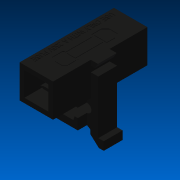
# Autodesk Inventor part: Soanar Power Module Fuse Cover
Saved by Autodesk Inventor 2016 (Build 200138000, 138)
## iProperties
Created: 2013-08-06
Material: ABS Plastic
Document SubType Name: Modeling
Designer: sdarley
Density: 1.06 g/cm^3
Appearance: Smooth - Black
Project: Power Entry Module - Soanar PP4003
Description: Soanar Power Module Fuse Cover
Author: sdarley
Title: Soanar Power Module Fuse Cover
Revision Number: 1
Autodesk Inventor part; units mm, degrees
ref_plane "YZ Plane" through (0, 0, 0) normal (1, 0, 0) x (0, 1, 0)
ref_plane "XZ Plane" through (0, 0, 0) normal (0, 1, 0) x (-1, 0, 0)
ref_plane "XY Plane" through (0, 0, 0) normal (0, 0, 1) x (1, 0, 0)
sketch "Sketch1" plane through (0, 0, 0) normal (0, 0, 1) x (1, 0, 0)
  line L0 (-3.05, -3.0141) -> (3.05, -3.0141)
  line L1 (3.05, 3.0141) -> (-3.05, 3.0141)
  line L2 (-3.05, 3.0141) -> (-3.05, -3.0141)
  line L3 (-3.05, -3.0141) -> (3.05, 3.0141) construction
  line L4 (3.05, -3.0141) -> (-3.05, 3.0141) construction
  line L5 (-4.25, -4.2) -> (4.25, -4.2)
  line L6 (4.25, -4.2) -> (4.25, 4.2)
  line L7 (4.25, 4.2) -> (-4.25, 4.2)
  line L8 (-4.25, 4.2) -> (-4.25, -4.2)
  line L9 (-4.25, -4.2) -> (4.25, 4.2) construction
  line L10 (4.25, -4.2) -> (-4.25, 4.2) construction
  line L11 (3.05, 1.3359) -> (2.2, 1.3359)
  line L12 (3.05, 1.9859) -> (2.2, 1.9859)
  arc A0 (2.2, 1.9859) -> (0.95, 1.6609) centre (2.2, -0.5805) ccw
  arc A1 (0.95, 1.6609) -> (2.2, 1.3359) centre (2.2, 3.9022) ccw
  line L13 (3.05, -3.0141) -> (3.05, 1.3359)
  line L14 (3.05, 1.9859) -> (3.05, 3.0141)
  point P0 (0, 0)
  dimension "d0" = 8.5
  dimension "d1" = 8.4
  dimension "d2" = 6.1
  dimension "d3" = 4.35
  dimension "d4" = 0.65
  dimension "d5" = 2.1
  dimension "d6" = 0.85
  constraints: 30 end point, 6 parallel, 5 perpendicular, 4 midpoint, 4 point on circle, 2 centre point, 2 horizontal, 2 tangent, 2 vertical alignment, 1 equal radius, 1 point on line
  measures "d0" distance between parallel lines of L6 L8
  measures "d1" distance between parallel lines of L5 L7
  measures "d2" distance between parallel lines of L13 L2
  measures "d3" distance between parallel lines of L0 L11
  measures "d4" distance between parallel lines of L11 L12
  measures "d5" distance from line of A0.end L14
  measures "d6" distance of L11.start L11.end
extrude "Extrusion1" add sketch "Sketch1" along normal mid plane 24
sketch "Sketch2" plane through (0, 0, 0) normal (0, 0, 1) x (1, 0, 0)
  line L0 (-3.05, 3.0141) -> (-3.05, -3.0141) projected
  line L1 (-3.05, -3.0141) -> (3.05, -3.0141) projected
  line L2 (3.05, -3.0141) -> (3.05, 1.3359) projected
  line L3 (3.05, 1.3359) -> (2.2, 1.3359) projected
  arc A0 (0.95, 1.6609) -> (2.2, 1.3359) centre (2.2, 3.9022) ccw projected
  arc A1 (2.2, 1.9859) -> (0.95, 1.6609) centre (2.2, -0.5805) ccw projected
  line L4 (2.2, 1.9859) -> (3.05, 1.9859) projected
  line L5 (3.05, 1.9859) -> (3.05, 3.0141) projected
  line L6 (3.05, 3.0141) -> (-3.05, 3.0141) projected
  line L7 (4.25, -4.2) -> (-4.25, -4.2) projected
  line L8 (-4.25, -4.2) -> (-4.25, 4.2) projected
  line L9 (-4.25, 4.2) -> (4.25, 4.2) projected
  line L10 (4.25, 4.2) -> (4.25, -4.2) projected
  line L11 (4.25, 1.45) -> (6.15, 1.45)
  line L12 (6.15, 1.45) -> (6.15, -12.1)
  line L13 (6.15, -12.1) -> (7.55, -12.1)
  line L14 (7.55, -12.1) -> (7.55, -14.2)
  line L15 (7.55, -14.2) -> (6.3, -14.2)
  line L16 (6.3, -14.2) -> (4.15, -12.25)
  line L17 (4.15, -12.25) -> (4.15, -11.2)
  line L18 (4.15, -11.2) -> (3.35, -10.7)
  line L19 (3.35, -10.7) -> (-4.25, -10.7)
  line L20 (-4.25, -10.7) -> (-4.25, -9.15)
  line L21 (-4.25, -9.15) -> (-1.15, -8.65)
  line L22 (-1.15, -8.65) -> (-1.15, -9)
  line L23 (-1.15, -9) -> (2.1, -9)
  line L24 (2.1, -9) -> (2.45, -8)
  line L25 (2.45, -8) -> (3.25, -8)
  arc A2 (3.25, -8) -> (3.25, -5.7) centre (3.25, -6.85) ccw
  line L26 (3.25, -5.7) -> (2.45, -5.7)
  arc A3 (2.45, -5.7) -> (1.8, -5.05) centre (1.8, -5.7) ccw
  line L27 (1.8, -5.05) -> (-1.15, -5.05)
  line L28 (-1.15, -5.05) -> (-1.15, -5.9)
  line L29 (-1.15, -5.9) -> (-4.25, -5)
  line L30 (-4.25, -5) -> (-4.25, -4.2)
  line L31 (-4.25, -4.2) -> (4.25, -4.2)
  line L32 (4.25, 1.45) -> (4.25, -4.2)
  line L33 (4.25, 4.2) -> (6.05, 4.2)
  line L34 (6.05, 4.2) -> (5.25, 2.85)
  line L35 (5.25, 2.85) -> (4.25, 2.85)
  line L36 (4.25, 4.2) -> (4.25, 2.85)
  point P0 (0, 0)
  dimension "d13" = 15.65
  dimension "d14" = 2.1
  dimension "d15" = 10.4
  dimension "d16" = 3.4
  dimension "d17" = 2
  dimension "d18" = 1.95
  dimension "d19" = 1.55
  dimension "d20" = 0.5
  dimension "d21" = 1.55
  dimension "d22" = 2.15
  dimension "d23" = 0.8
  dimension "d24" = 11.8
  dimension "d25" = 3.1
  dimension "d26" = 1.7
  dimension "d27" = 2.05
  dimension "d28" = 1.75
  dimension "d29" = 3.25
  dimension "d30" = 1
  dimension "d31" = 0.8
  dimension "d32" = 3.1
  dimension "d33" = 1.7
  dimension "d34" = 9.25
  dimension "d35" = 3.6
  dimension "d36" = 2.3
  dimension "d39" = 2.75
  dimension "d40" = 1.8
  dimension "d41" = 1
  dimension "d42" = 1.35
  constraints: 52 end point, 11 parallel, 4 perpendicular, 4 point on circle, 3 collinear, 2 centre point, 2 point on line, 2 tangent, 2 vertical alignment, 1 line through centre, 1 vertical
  measures "d13" distance between parallel lines of L15 L11
  measures "d14" distance between parallel lines of L15 L13
  measures "d15" distance between parallel lines of L8 L12
  measures "d16" distance between parallel lines of L14 L17
  measures "d17" distance between parallel lines of L12 L17
  measures "d18" distance from line of L16.end L15
  measures "d19" distance from line of L16.end L19
  measures "d20" distance from line of L17.end L19
  measures "d21" distance of L19.end L20.end
  measures "d22" distance from line of L15.end L17
  measures "d23" distance from line of L18.end L17
  measures "d24" distance between parallel lines of L14 L20
  measures "d25" distance from line of L21.end L20
  measures "d26" distance between parallel lines of L19 L23
  measures "d27" distance from line of L19 L21.end
  measures "d28" distance edge to line of A2 L12
  measures "d29" distance of L22.end L23.end
  measures "d30" distance between parallel lines of L23 L25
  measures "d31" distance from line of L29.end L7
  measures "d32" distance from line of L28.end L30
  measures "d33" distance from line of L7 L28.end
  measures "d34" distance between parallel lines of L9 L27
  measures "d35" horizontal distance of L28.end L26.end
  measures "d36" distance between parallel lines of L25 L26
  measures "d39" distance between parallel lines of L9 L11
  measures "d40" distance of L9.end L33.end
  measures "d41" distance of L34.end L35.end
  measures "d42" distance between parallel lines of L35 L33
extrude "Extrusion2" add sketch "Sketch2" along normal mid plane 4.8
sketch "Sketch3" plane through (0, 0, 2.4) normal (0, 0, 1) x (1, 0, 0)
  line L0 (-4.25, -4.2) -> (4.25, -4.2) projected
  line L1 (-4.25, -4.2) -> (-4.25, -5) projected
  line L2 (-4.25, -5) -> (-1.15, -5.9) projected
  line L3 (-1.15, -5.9) -> (-1.15, -5.05) projected
  line L4 (-1.15, -5.05) -> (1.8, -5.05) projected
  arc A0 (2.45, -5.7) -> (1.8, -5.05) centre (1.8, -5.7) ccw projected
  line L5 (2.45, -5.7) -> (3.25, -5.7) projected
  line L6 (3.25, -8) -> (2.45, -8) projected
  line L7 (2.45, -8) -> (2.1, -9) projected
  line L8 (2.1, -9) -> (-1.15, -9) projected
  line L9 (-1.15, -9) -> (-1.15, -8.65) projected
  line L10 (-1.15, -8.65) -> (-4.25, -9.15) projected
  line L11 (-4.25, -9.15) -> (-4.25, -10.7) projected
  line L12 (-4.25, -10.7) -> (3.35, -10.7) projected
  line L13 (3.25, -4.2) -> (3.25, -5.7)
  line L14 (3.25, -8) -> (3.25, -10.7)
  point P0 (0, 0)
  dimension "d43" = 7.5
  constraints: 4 end point, 4 point on line, 2 perpendicular, 1 vertical alignment
  measures "d43" distance between parallel lines of L14 L11
extrude "Extrusion3" add sketch "Sketch3" along normal blind 2.3
sketch "Sketch4" plane through (0, 0, -2.4) normal (0, 0, -1) x (-1, 0, 0)
  line L0 (-3.35, -10.7) -> (4.25, -10.7) projected
  line L1 (4.25, -10.7) -> (4.25, -9.15) projected
  line L2 (4.25, -9.15) -> (1.15, -8.65) projected
  line L3 (1.15, -8.65) -> (1.15, -9) projected
  line L4 (1.15, -9) -> (-2.1, -9) projected
  line L5 (-2.1, -9) -> (-2.45, -8) projected
  line L6 (-2.45, -8) -> (-3.25, -8) projected
  line L7 (-3.25, -5.7) -> (-2.45, -5.7) projected
  arc A0 (-1.8, -5.05) -> (-2.45, -5.7) centre (-1.8, -5.7) ccw projected
  line L8 (-1.8, -5.05) -> (1.15, -5.05) projected
  line L9 (1.15, -5.05) -> (1.15, -5.9) projected
  line L10 (1.15, -5.9) -> (4.25, -5) projected
  line L11 (4.25, -5) -> (4.25, -4.2) projected
  line L12 (-4.25, -4.2) -> (4.25, -4.2) projected
  line L13 (-3.25, -4.2) -> (-3.25, -5.7) projected
  line L14 (-3.25, -8) -> (-3.25, -10.7) projected
  point P0 (0, 0)
extrude "Extrusion4" add sketch "Sketch4" along normal blind 2.3
sketch "Sketch8" plane through (-4.25, 4.2, -12) normal (0, 1, 0) x (1, 0, 0)
  line L0 (8.5, 0) -> (8.5, -9.6) projected
  line L1 (0, 0) -> (8.5, 0) projected
  line L2 (6.575, -9.05) -> (6.575, -15.85)
  line L3 (3.575, -15.85) -> (3.575, -9.05)
  arc A0 (3, -8.475) -> (3.575, -9.05) centre (3.575, -8.475) ccw
  arc A1 (6.575, -9.05) -> (7.15, -8.475) centre (6.575, -8.475) ccw
  line L4 (3, -8.475) -> (3, -6.225)
  line L5 (3, -6.225) -> (4.025, -5.2)
  line L6 (4.025, -5.2) -> (6.125, -5.2)
  line L7 (6.125, -5.2) -> (7.15, -6.225)
  line L8 (7.15, -6.225) -> (7.15, -8.475)
  line L9 (3, -16.425) -> (3, -18.675)
  line L10 (3, -18.675) -> (4.025, -19.7)
  line L11 (4.025, -19.7) -> (6.125, -19.7)
  line L12 (6.125, -19.7) -> (7.15, -18.675)
  line L13 (7.15, -18.675) -> (7.15, -16.425)
  arc A2 (3.575, -15.85) -> (3, -16.425) centre (3.575, -16.425) ccw
  arc A3 (7.15, -16.425) -> (6.575, -15.85) centre (6.575, -16.425) ccw
  line L14 (4.025, -8.95) -> (6.125, -8.95)
  line L15 (6.125, -8.95) -> (6.125, -15.95)
  line L16 (6.125, -15.95) -> (4.025, -15.95)
  line L17 (4.025, -15.95) -> (4.025, -8.95)
  line L18 (4.2114, -5.65) -> (5.9386, -5.65)
  line L19 (5.9386, -5.65) -> (6.7, -6.4114)
  line L20 (6.7, -6.4114) -> (6.7, -8.5)
  line L21 (6.7, -8.5) -> (3.45, -8.5)
  line L22 (3.45, -8.5) -> (3.45, -6.4114)
  line L23 (3.45, -6.4114) -> (4.2114, -5.65)
  line L24 (3.45, -18.4886) -> (3.45, -16.4)
  line L25 (3.45, -16.4) -> (6.7, -16.4)
  line L26 (6.7, -16.4) -> (6.7, -18.4886)
  line L27 (6.7, -18.4886) -> (5.9386, -19.25)
  line L28 (5.9386, -19.25) -> (4.2114, -19.25)
  line L29 (4.2114, -19.25) -> (3.45, -18.4886)
  point P0 (4.25, -12)
  point P1 (5.075, -5.2)
  point P2 (5.075, -19.7)
  point P3 (5.075, -5.65)
  point P4 (5.075, -8.5)
  point P5 (5.075, -16.4)
  point P6 (5.075, -19.25)
  dimension "d90" = 14.5
  dimension "d91" = 1.35
  dimension "d92" = 4.15
  dimension "d93" = 3
  dimension "d95" = 6.8
  dimension "d96" = 2.1
  dimension "d97" = 5.2
  dimension "d104" = 7
  dimension "d105" = 0.45
  dimension "d106" = 0.45
  dimension "d107" = 0.45
  dimension "d108" = 0.45
  dimension "d109" = 0.45
  dimension "d110" = 0.45
  dimension "d111" = 0.45
  dimension "d112" = 0.45
  dimension "d113" = 0.45
  dimension "d114" = 0.45
  constraints: 56 end point, 16 parallel, 9 perpendicular, 8 point on circle, 7 vertical alignment, 6 midpoint, 5 horizontal alignment, 4 centre point, 4 equal length, 4 line through centre, 3 tangent, 1 collinear, 1 equal radius, 1 horizontal, 1 vertical
  measures "d90" distance between parallel lines of L11 L6
  measures "d91" distance between parallel lines of L0 L8
  measures "d92" distance between parallel lines of L8 L4
  measures "d93" distance between parallel lines of L2 L3
  measures "d95" distance of L3.start L3.end
  measures "d96" distance of L5.end L6.end
  measures "d97" distance between parallel lines of L1 L6
  measures "d104" distance between parallel lines of L16 L14
  measures "d105" distance between parallel lines of L2 L15
  measures "d106" distance between parallel lines of L17 L3
  measures "d107" distance between parallel lines of L5 L23
  measures "d108" distance between parallel lines of L8 L20
  measures "d109" distance between parallel lines of L6 L18
  measures "d110" distance between parallel lines of L21 L14
  measures "d111" distance between parallel lines of L11 L28
  measures "d112" distance between parallel lines of L13 L26
  measures "d113" distance between parallel lines of L12 L27
  measures "d114" distance between parallel lines of L16 L25
extrude "Extrusion8" cut sketch "Sketch8" against normal blind 0.1
sketch "Sketch5" plane through (-4.25, 4.2, -12) normal (0, 1, 0) x (1, 0, 0)
  line L0 (0, 0) -> (0, -24) projected
  line L1 (1.85, -1.3407) -> (1.85, -22.6593) construction
  line L2 (1.85, -22.6593) -> (0.5, -22.6593) construction
  line L3 (0.5, -22.6593) -> (0.5, -1.3407) construction
  line L4 (0.5, -1.3407) -> (1.85, -1.3407) construction
  line L5 (1.8278, -2.1206) -> (1.8278, -2.2557)
  line L6 (1.8278, -2.2557) -> (1.1058, -2.2557)
  spline S0 degree 2 poles (1.1058, -2.2557) (0.9243, -2.2557) (0.6917, -2.1853) (0.5566, -1.999) (0.5566, -1.8551) knots 0 0 0 1 2 3 3 3
  spline S1 degree 2 poles (0.5566, -1.8551) (0.5566, -1.6524) (0.7988, -1.4507) (1.1058, -1.4507) knots 0 0 0 1 2 2 2
  line L7 (1.1058, -1.4507) -> (1.8278, -1.4507)
  line L8 (1.8278, -1.4507) -> (1.8278, -1.5858)
  line L9 (1.8278, -1.5858) -> (1.1068, -1.5858)
  spline S2 degree 2 poles (1.1068, -1.5858) (0.9369, -1.5858) (0.7853, -1.6389) (0.7062, -1.7586) (0.7062, -1.8455) knots 0 0 0 1 2 3 3 3
  spline S3 degree 2 poles (0.7062, -1.8455) (0.7062, -1.9903) (0.8703, -2.1206) (1.1068, -2.1206) knots 0 0 0 1 2 2 2
  line L10 (1.1068, -2.1206) -> (1.8278, -2.1206)
  line L11 (0.9803, -2.4391) -> (0.9938, -2.5675)
  spline S4 degree 2 poles (0.9938, -2.5675) (0.8905, -2.5781) (0.7757, -2.6505) (0.7062, -2.7847) (0.7062, -2.8696) knots 0 0 0 1 2 3 3 3
  spline S5 degree 2 poles (0.7062, -2.8696) (0.7062, -2.9903) (0.8239, -3.1244) (0.9185, -3.1244) knots 0 0 0 1 2 2 2
  spline S6 degree 2 poles (0.9185, -3.1244) (0.9736, -3.1244) (1.0556, -3.0762) (1.1087, -2.9777) (1.1569, -2.8146) knots 0 0 0 1 2 3 3 3
  spline S7 degree 2 poles (1.1569, -2.8146) (1.2004, -2.6698) (1.2873, -2.5472) (1.4214, -2.4787) (1.5054, -2.4787) knots 0 0 0 1 2 3 3 3
  spline S8 degree 2 poles (1.5054, -2.4787) (1.6569, -2.4787) (1.85, -2.6746) (1.85, -2.8407) knots 0 0 0 1 2 2 2
  spline S9 degree 2 poles (1.85, -2.8407) (1.85, -2.9555) (1.7593, -3.1264) (1.5903, -3.221) (1.4764, -3.2248) knots 0 0 0 1 2 3 3 3
  line L12 (1.4764, -3.2248) -> (1.4649, -3.0945)
  spline S10 degree 2 poles (1.4649, -3.0945) (1.5865, -3.0839) (1.7042, -2.9584) (1.7042, -2.8455) knots 0 0 0 1 2 2 2
  spline S11 degree 2 poles (1.7042, -2.8455) (1.7042, -2.7306) (1.601, -2.609) (1.5189, -2.609) knots 0 0 0 1 2 2 2
  spline S12 degree 2 poles (1.5189, -2.609) (1.4436, -2.609) (1.4021, -2.6534) knots 0 0 0 1 1 1
  spline S13 degree 2 poles (1.4021, -2.6534) (1.3597, -2.6978) (1.3172, -2.8532) knots 0 0 0 1 1 1
  spline S14 degree 2 poles (1.3172, -2.8532) (1.2747, -3.0047) (1.2438, -3.0665) knots 0 0 0 1 1 1
  spline S15 degree 2 poles (1.2438, -3.0665) (1.1965, -3.1602) (1.0402, -3.2557) (0.932, -3.2557) knots 0 0 0 1 2 2 2
  spline S16 degree 2 poles (0.932, -3.2557) (0.8249, -3.2557) (0.6483, -3.1553) (0.5566, -2.9816) (0.5566, -2.86) knots 0 0 0 1 2 3 3 3
  spline S17 degree 2 poles (0.5566, -2.86) (0.5566, -2.6698) (0.7853, -2.443) (0.9803, -2.4391) knots 0 0 0 1 2 2 2
  line L13 (0.5778, -3.442) -> (1.8278, -3.442)
  line L14 (1.8278, -3.442) -> (1.8278, -4.1824)
  line L15 (1.8278, -4.1824) -> (1.6801, -4.1824)
  line L16 (1.6801, -4.1824) -> (1.6801, -3.5771)
  line L17 (1.6801, -3.5771) -> (1.2988, -3.5771)
  line L18 (1.2988, -3.5771) -> (1.2988, -4.1437)
  line L19 (1.2988, -4.1437) -> (1.1512, -4.1437)
  line L20 (1.1512, -4.1437) -> (1.1512, -3.5771)
  line L21 (1.1512, -3.5771) -> (0.7255, -3.5771)
  line L22 (0.7255, -3.5771) -> (0.7255, -4.2065)
  line L23 (0.7255, -4.2065) -> (0.5778, -4.2065)
  line L24 (0.5778, -4.2065) -> (0.5778, -3.442)
  spline S18 degree 2 poles (1.1869, -4.7547) (1.5064, -4.7547) (1.85, -5.0366) (1.85, -5.2461) knots 0 0 0 1 2 2 2
  spline S19 degree 2 poles (1.85, -5.2461) (1.85, -5.3812) (1.6965, -5.6051) (1.4041, -5.7354) (1.2023, -5.7354) knots 0 0 0 1 2 3 3 3
  spline S20 degree 2 poles (1.2023, -5.7354) (0.9243, -5.7354) (0.7496, -5.609) knots 0 0 0 1 1 1
  spline S21 degree 2 poles (0.7496, -5.609) (0.5566, -5.47) (0.5566, -5.2451) knots 0 0 0 1 1 1
  spline S22 degree 2 poles (0.5566, -5.2451) (0.5566, -5.0183) (0.7544, -4.8802) knots 0 0 0 1 1 1
  spline S23 degree 2 poles (0.7544, -4.8802) (0.933, -4.7547) (1.1869, -4.7547) knots 0 0 0 1 1 1
  spline S24 degree 2 poles (1.1849, -4.8937) (0.9533, -4.8937) (0.6985, -5.0984) (0.6985, -5.2441) knots 0 0 0 1 2 2 2
  spline S25 degree 2 poles (0.6985, -5.2441) (0.6985, -5.3937) (0.9562, -5.5964) (1.2062, -5.5964) knots 0 0 0 1 2 2 2
  spline S26 degree 2 poles (1.2062, -5.5964) (1.3674, -5.5964) (1.4938, -5.5443) knots 0 0 0 1 1 1
  spline S27 degree 2 poles (1.4938, -5.5443) (1.5913, -5.5038) (1.7081, -5.3426) (1.7081, -5.247) knots 0 0 0 1 2 2 2
  spline S28 degree 2 poles (1.7081, -5.247) (1.7081, -5.0926) (1.4523, -4.8937) (1.1849, -4.8937) knots 0 0 0 1 2 2 2
  line L25 (0.5778, -5.9024) -> (1.8278, -5.9024)
  line L26 (1.8278, -5.9024) -> (1.8278, -6.0414)
  line L27 (1.8278, -6.0414) -> (0.8461, -6.58)
  line L28 (0.8461, -6.58) -> (1.8278, -6.58)
  line L29 (1.8278, -6.58) -> (1.8278, -6.7094)
  line L30 (1.8278, -6.7094) -> (0.5778, -6.7094)
  line L31 (0.5778, -6.7094) -> (0.5778, -6.5704)
  line L32 (0.5778, -6.5704) -> (1.5575, -6.0327)
  line L33 (1.5575, -6.0327) -> (0.5778, -6.0327)
  line L34 (0.5778, -6.0327) -> (0.5778, -5.9024)
  line L35 (0.5778, -6.9324) -> (1.8278, -6.9324)
  line L36 (1.8278, -6.9324) -> (1.8278, -7.0675)
  line L37 (1.8278, -7.0675) -> (0.7255, -7.0675)
  line L38 (0.7255, -7.0675) -> (0.7255, -7.5723)
  line L39 (0.7255, -7.5723) -> (0.5778, -7.5723)
  line L40 (0.5778, -7.5723) -> (0.5778, -6.9324)
  line L41 (0.5778, -8.025) -> (1.1077, -8.025)
  line L42 (1.1077, -8.025) -> (1.8278, -7.6302)
  line L43 (1.8278, -7.6302) -> (1.8278, -7.7963)
  line L44 (1.8278, -7.7963) -> (1.4514, -7.997)
  spline S29 degree 2 poles (1.4514, -7.997) (1.3403, -8.0559) (1.24, -8.1013) knots 0 0 0 1 1 1
  spline S30 degree 2 poles (1.24, -8.1013) (1.3384, -8.1466) (1.461, -8.2132) knots 0 0 0 1 1 1
  line L45 (1.461, -8.2132) -> (1.8278, -8.4121)
  line L46 (1.8278, -8.4121) -> (1.8278, -8.5694)
  line L47 (1.8278, -8.5694) -> (1.1077, -8.1602)
  line L48 (1.1077, -8.1602) -> (0.5778, -8.1602)
  line L49 (0.5778, -8.1602) -> (0.5778, -8.025)
  line L50 (0.5778, -9.2712) -> (1.8278, -8.999)
  line L51 (1.8278, -8.999) -> (1.8278, -9.138)
  line L52 (1.8278, -9.138) -> (1.0083, -9.2934)
  spline S31 degree 2 poles (1.0083, -9.2934) (0.8819, -9.3185) (0.7525, -9.3378) knots 0 0 0 1 1 1
  line L53 (0.7525, -9.3378) -> (0.9832, -9.3831)
  line L54 (0.9832, -9.3831) -> (1.8278, -9.5791)
  line L55 (1.8278, -9.5791) -> (1.8278, -9.7422)
  line L56 (1.8278, -9.7422) -> (1.1956, -9.8889)
  spline S32 degree 2 poles (1.1956, -9.8889) (0.9639, -9.942) (0.7525, -9.969) knots 0 0 0 1 1 1
  spline S33 degree 2 poles (0.7525, -9.969) (0.8741, -9.9883) (1.0247, -10.0192) knots 0 0 0 1 1 1
  line L57 (1.0247, -10.0192) -> (1.8278, -10.1804)
  line L58 (1.8278, -10.1804) -> (1.8278, -10.3175)
  line L59 (1.8278, -10.3175) -> (0.5778, -10.0366)
  line L60 (0.5778, -10.0366) -> (0.5778, -9.9044)
  line L61 (0.5778, -9.9044) -> (1.5305, -9.6881)
  line L62 (1.5305, -9.6881) -> (1.6772, -9.6563)
  spline S34 degree 2 poles (1.6772, -9.6563) (1.5952, -9.6418) (1.5305, -9.6264) knots 0 0 0 1 1 1
  line L63 (1.5305, -9.6264) -> (0.5778, -9.4092)
  line L64 (0.5778, -9.4092) -> (0.5778, -9.2712)
  line L65 (0.5778, -10.4681) -> (1.8278, -10.4681)
  line L66 (1.8278, -10.4681) -> (1.8278, -10.6032)
  line L67 (1.8278, -10.6032) -> (0.5778, -10.6032)
  line L68 (0.5778, -10.6032) -> (0.5778, -10.4681)
  line L69 (0.5778, -11.1032) -> (1.6801, -11.1032)
  line L70 (1.6801, -11.1032) -> (1.6801, -10.7654)
  line L71 (1.6801, -10.7654) -> (1.8278, -10.7654)
  line L72 (1.8278, -10.7654) -> (1.8278, -11.5781)
  line L73 (1.8278, -11.5781) -> (1.6801, -11.5781)
  line L74 (1.6801, -11.5781) -> (1.6801, -11.2383)
  line L75 (1.6801, -11.2383) -> (0.5778, -11.2383)
  line L76 (0.5778, -11.2383) -> (0.5778, -11.1032)
  line L77 (0.5778, -11.7142) -> (1.8278, -11.7142)
  line L78 (1.8278, -11.7142) -> (1.8278, -11.8493)
  line L79 (1.8278, -11.8493) -> (1.3143, -11.8493)
  line L80 (1.3143, -11.8493) -> (1.3143, -12.3831)
  line L81 (1.3143, -12.3831) -> (1.8278, -12.3831)
  line L82 (1.8278, -12.3831) -> (1.8278, -12.5183)
  line L83 (1.8278, -12.5183) -> (0.5778, -12.5183)
  line L84 (0.5778, -12.5183) -> (0.5778, -12.3831)
  line L85 (0.5778, -12.3831) -> (1.1666, -12.3831)
  line L86 (1.1666, -12.3831) -> (1.1666, -11.8493)
  line L87 (1.1666, -11.8493) -> (0.5778, -11.8493)
  line L88 (0.5778, -11.8493) -> (0.5778, -11.7142)
  line L89 (0.5778, -13.0347) -> (1.8278, -13.4285)
  line L90 (1.8278, -13.4285) -> (1.8278, -13.5752)
  line L91 (1.8278, -13.5752) -> (0.5778, -13.9941)
  line L92 (0.5778, -13.9941) -> (0.5778, -13.8387)
  line L93 (0.5778, -13.8387) -> (0.9562, -13.72)
  line L94 (0.9562, -13.72) -> (0.9562, -13.2895)
  line L95 (0.9562, -13.2895) -> (0.5778, -13.1785)
  line L96 (0.5778, -13.1785) -> (0.5778, -13.0347)
  line L97 (1.0913, -13.3291) -> (1.0913, -13.6775)
  line L98 (1.0913, -13.6775) -> (1.4378, -13.5714)
  spline S35 degree 2 poles (1.4378, -13.5714) (1.5971, -13.5212) (1.6965, -13.499) knots 0 0 0 1 1 1
  spline S36 degree 2 poles (1.6965, -13.499) (1.5759, -13.4787) (1.4581, -13.443) knots 0 0 0 1 1 1
  line L99 (1.4581, -13.443) -> (1.0913, -13.3291)
  line L100 (0.7255, -15.11) -> (0.5778, -15.11)
  line L101 (0.5778, -15.11) -> (0.5778, -14.4324)
  spline S37 degree 2 poles (0.5778, -14.4324) (0.6676, -14.4295) (0.8896, -14.5434) (1.0402, -14.6939) knots 0 0 0 1 2 2 2
  spline S38 degree 2 poles (1.0402, -14.6939) (1.2158, -14.8696) (1.4079, -14.9787) (1.49, -14.9787) knots 0 0 0 1 2 2 2
  spline S39 degree 2 poles (1.49, -14.9787) (1.5855, -14.9787) (1.7062, -14.8677) (1.7062, -14.7856) knots 0 0 0 1 2 2 2
  spline S40 degree 2 poles (1.7062, -14.7856) (1.7062, -14.6978) (1.5759, -14.5858) (1.4542, -14.5858) knots 0 0 0 1 2 2 2
  line L102 (1.4542, -14.5858) -> (1.4707, -14.4565)
  spline S41 degree 2 poles (1.4707, -14.4565) (1.6512, -14.47) (1.8326, -14.6466) (1.8326, -14.7905) knots 0 0 0 1 2 2 2
  spline S42 degree 2 poles (1.8326, -14.7905) (1.8326, -14.9468) (1.6212, -15.108) (1.4871, -15.108) knots 0 0 0 1 2 2 2
  spline S43 degree 2 poles (1.4871, -15.108) (1.3674, -15.108) (1.1483, -14.9816) (0.9658, -14.8059) knots 0 0 0 1 2 2 2
  spline S44 degree 2 poles (0.9658, -14.8059) (0.851, -14.693) (0.767, -14.6273) (0.7255, -14.6071) knots 0 0 0 1 2 2 2
  line L103 (0.7255, -14.6071) -> (0.7255, -15.11)
  line L104 (0.905, -15.2432) -> (0.9185, -15.3754)
  spline S45 degree 2 poles (0.9185, -15.3754) (0.7998, -15.3908) (0.683, -15.499) (0.683, -15.5704) knots 0 0 0 1 2 2 2
  spline S46 degree 2 poles (0.683, -15.5704) (0.683, -15.6602) (0.8481, -15.7895) (0.99, -15.7895) knots 0 0 0 1 2 2 2
  spline S47 degree 2 poles (0.99, -15.7895) (1.1241, -15.7895) (1.2718, -15.664) (1.2718, -15.5694) knots 0 0 0 1 2 2 2
  spline S48 degree 2 poles (1.2718, -15.5694) (1.2718, -15.5125) (1.2081, -15.4131) (1.1502, -15.3841) knots 0 0 0 1 2 2 2
  line L105 (1.1502, -15.3841) -> (1.1695, -15.2654)
  line L106 (1.1695, -15.2654) -> (1.8114, -15.3648)
  line L107 (1.8114, -15.3648) -> (1.8114, -15.8744)
  line L108 (1.8114, -15.8744) -> (1.6647, -15.8744)
  line L109 (1.6647, -15.8744) -> (1.6647, -15.4642)
  line L110 (1.6647, -15.4642) -> (1.3288, -15.4102)
  spline S49 degree 2 poles (1.3288, -15.4102) (1.4069, -15.5019) (1.4069, -15.6042) knots 0 0 0 1 1 1
  spline S50 degree 2 poles (1.4069, -15.6042) (1.4069, -15.7325) (1.1878, -15.9227) (1.0015, -15.9227) knots 0 0 0 1 2 2 2
  spline S51 degree 2 poles (1.0015, -15.9227) (0.8181, -15.9227) (0.5566, -15.7325) (0.5566, -15.5723) knots 0 0 0 1 2 2 2
  spline S52 degree 2 poles (0.5566, -15.5723) (0.5566, -15.4391) (0.7419, -15.2557) (0.905, -15.2432) knots 0 0 0 1 2 2 2
  spline S53 degree 2 poles (1.1946, -16.0395) (1.5083, -16.0395) (1.8326, -16.2094) (1.8326, -16.3744) knots 0 0 0 1 2 2 2
  spline S54 degree 2 poles (1.8326, -16.3744) (1.8326, -16.5212) (1.7014, -16.6061) knots 0 0 0 1 1 1
  spline S55 degree 2 poles (1.7014, -16.6061) (1.5431, -16.7084) (1.1946, -16.7084) knots 0 0 0 1 1 1
  spline S56 degree 2 poles (1.1946, -16.7084) (0.8809, -16.7084) (0.5566, -16.5395) (0.5566, -16.3735) knots 0 0 0 1 2 2 2
  spline S57 degree 2 poles (0.5566, -16.3735) (0.5566, -16.2268) (0.8432, -16.0395) (1.1946, -16.0395) knots 0 0 0 1 2 2 2
  spline S58 degree 2 poles (1.1946, -16.1688) (0.8905, -16.1688) (0.683, -16.2856) (0.683, -16.3773) knots 0 0 0 1 2 2 2
  spline S59 degree 2 poles (0.683, -16.3773) (0.683, -16.4632) (0.8925, -16.5791) (1.1946, -16.5791) knots 0 0 0 1 2 2 2
  spline S60 degree 2 poles (1.1946, -16.5791) (1.4996, -16.5791) (1.7062, -16.4623) (1.7062, -16.3696) knots 0 0 0 1 2 2 2
  spline S61 degree 2 poles (1.7062, -16.3696) (1.7062, -16.2837) (1.4967, -16.1688) (1.1946, -16.1688) knots 0 0 0 1 2 2 2
  line L111 (0.5778, -17.1833) -> (1.8278, -16.7856)
  line L112 (1.8278, -16.7856) -> (1.8278, -16.9324)
  line L113 (1.8278, -16.9324) -> (0.9195, -17.1997)
  spline S62 degree 2 poles (0.9195, -17.1997) (0.8143, -17.2306) (0.7149, -17.2538) knots 0 0 0 1 1 1
  spline S63 degree 2 poles (0.7149, -17.2538) (0.8181, -17.277) (0.9195, -17.3078) knots 0 0 0 1 1 1
  line L114 (0.9195, -17.3078) -> (1.8278, -17.5849)
  line L115 (1.8278, -17.5849) -> (1.8278, -17.7229)
  line L116 (1.8278, -17.7229) -> (0.5778, -17.3233)
  line L117 (0.5778, -17.3233) -> (0.5778, -17.1833)
  line L118 (0.5778, -18.2528) -> (1.8278, -18.2528)
  line L119 (1.8278, -18.2528) -> (1.8278, -18.9439)
  line L120 (1.8278, -18.9439) -> (1.6801, -18.9439)
  line L121 (1.6801, -18.9439) -> (1.6801, -18.388)
  line L122 (1.6801, -18.388) -> (1.2931, -18.388)
  line L123 (1.2931, -18.388) -> (1.2931, -18.8686)
  line L124 (1.2931, -18.8686) -> (1.1454, -18.8686)
  line L125 (1.1454, -18.8686) -> (1.1454, -18.388)
  line L126 (1.1454, -18.388) -> (0.5778, -18.388)
  line L127 (0.5778, -18.388) -> (0.5778, -18.2528)
  line L128 (1.8278, -19.7866) -> (1.8278, -19.9217)
  line L129 (1.8278, -19.9217) -> (1.1058, -19.9217)
  spline S64 degree 2 poles (1.1058, -19.9217) (0.9243, -19.9217) (0.6917, -19.8513) (0.5566, -19.665) (0.5566, -19.5212) knots 0 0 0 1 2 3 3 3
  spline S65 degree 2 poles (0.5566, -19.5212) (0.5566, -19.3185) (0.7988, -19.1167) (1.1058, -19.1167) knots 0 0 0 1 2 2 2
  line L130 (1.1058, -19.1167) -> (1.8278, -19.1167)
  line L131 (1.8278, -19.1167) -> (1.8278, -19.2519)
  line L132 (1.8278, -19.2519) -> (1.1068, -19.2519)
  spline S66 degree 2 poles (1.1068, -19.2519) (0.9369, -19.2519) (0.7853, -19.3049) (0.7062, -19.4246) (0.7062, -19.5115) knots 0 0 0 1 2 3 3 3
  spline S67 degree 2 poles (0.7062, -19.5115) (0.7062, -19.6563) (0.8703, -19.7866) (1.1068, -19.7866) knots 0 0 0 1 2 2 2
  line L133 (1.1068, -19.7866) -> (1.8278, -19.7866)
  line L134 (0.9803, -20.1051) -> (0.9938, -20.2335)
  spline S68 degree 2 poles (0.9938, -20.2335) (0.8905, -20.2441) (0.7757, -20.3165) (0.7062, -20.4507) (0.7062, -20.5356) knots 0 0 0 1 2 3 3 3
  spline S69 degree 2 poles (0.7062, -20.5356) (0.7062, -20.6563) (0.8239, -20.7905) (0.9185, -20.7905) knots 0 0 0 1 2 2 2
  spline S70 degree 2 poles (0.9185, -20.7905) (0.9736, -20.7905) (1.0556, -20.7422) (1.1087, -20.6437) (1.1569, -20.4806) knots 0 0 0 1 2 3 3 3
  spline S71 degree 2 poles (1.1569, -20.4806) (1.2004, -20.3358) (1.2873, -20.2132) (1.4214, -20.1447) (1.5054, -20.1447) knots 0 0 0 1 2 3 3 3
  spline S72 degree 2 poles (1.5054, -20.1447) (1.6569, -20.1447) (1.85, -20.3407) (1.85, -20.5067) knots 0 0 0 1 2 2 2
  spline S73 degree 2 poles (1.85, -20.5067) (1.85, -20.6215) (1.7593, -20.7924) (1.5903, -20.887) (1.4764, -20.8908) knots 0 0 0 1 2 3 3 3
  line L135 (1.4764, -20.8908) -> (1.4649, -20.7605)
  spline S74 degree 2 poles (1.4649, -20.7605) (1.5865, -20.7499) (1.7042, -20.6244) (1.7042, -20.5115) knots 0 0 0 1 2 2 2
  spline S75 degree 2 poles (1.7042, -20.5115) (1.7042, -20.3966) (1.601, -20.275) (1.5189, -20.275) knots 0 0 0 1 2 2 2
  spline S76 degree 2 poles (1.5189, -20.275) (1.4436, -20.275) (1.4021, -20.3194) knots 0 0 0 1 1 1
  spline S77 degree 2 poles (1.4021, -20.3194) (1.3597, -20.3638) (1.3172, -20.5192) knots 0 0 0 1 1 1
  spline S78 degree 2 poles (1.3172, -20.5192) (1.2747, -20.6708) (1.2438, -20.7325) knots 0 0 0 1 1 1
  spline S79 degree 2 poles (1.2438, -20.7325) (1.1965, -20.8262) (1.0402, -20.9217) (0.932, -20.9217) knots 0 0 0 1 2 2 2
  spline S80 degree 2 poles (0.932, -20.9217) (0.8249, -20.9217) (0.6483, -20.8214) (0.5566, -20.6476) (0.5566, -20.526) knots 0 0 0 1 2 3 3 3
  spline S81 degree 2 poles (0.5566, -20.526) (0.5566, -20.3358) (0.7853, -20.109) (0.9803, -20.1051) knots 0 0 0 1 2 2 2
  line L136 (0.5778, -21.108) -> (1.8278, -21.108)
  line L137 (1.8278, -21.108) -> (1.8278, -21.8484)
  line L138 (1.8278, -21.8484) -> (1.6801, -21.8484)
  line L139 (1.6801, -21.8484) -> (1.6801, -21.2432)
  line L140 (1.6801, -21.2432) -> (1.2988, -21.2432)
  line L141 (1.2988, -21.2432) -> (1.2988, -21.8098)
  line L142 (1.2988, -21.8098) -> (1.1512, -21.8098)
  line L143 (1.1512, -21.8098) -> (1.1512, -21.2432)
  line L144 (1.1512, -21.2432) -> (0.7255, -21.2432)
  line L145 (0.7255, -21.2432) -> (0.7255, -21.8725)
  line L146 (0.7255, -21.8725) -> (0.5778, -21.8725)
  line L147 (0.5778, -21.8725) -> (0.5778, -21.108)
  point P0 (4.25, -12)
  point P1 (1.85, -12)
  dimension "d48" = 1.35
  dimension "d49" = 0.5
  constraints: 1 horizontal alignment, 1 midpoint, 1 vertical, 2 other
  measures "d48" distance between parallel lines of L1 L3
  measures "d49" distance between parallel lines of L0 L3
emboss "Emboss1" sketch "Sketch5" operation add depth 0.1 direction (0, -1, 0)
equation "\"d25\" = d32"
body "Solid1"
